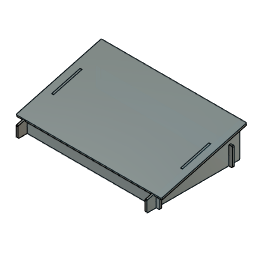
Laptop Stand (Autodesk Fusion 360 design; units mm, degrees)
Autodesk Fusion 360 part; units mm, degrees
sketch "Sketch1" plane through (0, 0, 0) normal (1, 0, 0) x (0, 1, 0) in component "Leg"
  line L0 (0, 0) -> (252.4348, 0)
  line L1 (252.4348, 0) -> (252.4348, 92.1166)
  line L2 (20.6126, 30) -> (19.3185, 34.8296)
  line L3 (19.3185, 34.8296) -> (0, 29.6532)
  line L4 (0, 29.6532) -> (0, 0)
  line L5 (97.8867, 50.7055) -> (96.5926, 55.5352)
  line L6 (96.5926, 55.5352) -> (173.8666, 76.2407)
  line L7 (173.8666, 76.2407) -> (175.1607, 71.411)
  line L8 (252.4348, 92.1166) -> (175.1607, 71.411)
  line L9 (97.8867, 50.7055) -> (20.6126, 30)
  dimension "d4" = 15
  dimension "d5" = 240
  dimension "d6" = 20
  dimension "d8" = 30
  dimension "d9" = 5
  dimension "d17" = 5
  dimension "d18" = 80
  dimension "d19" = 80
  constraint coincident L0.start L4.end
  constraint horizontal L0
  constraint perpendicular L0 L1
  constraint perpendicular L2 L8
  constraint perpendicular L0 L4
  constraint parallel L3 L8
  constraint coincident L5.start L8
  constraint perpendicular L5 L8
  constraint perpendicular L5 L6
  constraint perpendicular L7 L8
  constraint collinear L8 L9
  measures "d4" angle of L0 L8
  measures "d5" distance of L1.end L2.start
  measures "d6" distance of L2.end L3.end
  measures "d8" distance of L0 L2.start
  measures "d9" distance of L2.start L2.end
  measures "d17" distance of L5.start L5.end
  measures "d18" distance of L2 L5
  measures "d19" distance of L5.end L6.end
extrude "Extrude1" add sketch "Sketch1" along normal blind 5 makes body 1 in component "Leg"
sketch "Sketch1 (2)" plane through (0, -6.1192, 22.8372) normal (0, -0.258819, 0.965926) x (1, 0, 0) in component "Top"
  line L0 (0, 107.6748) -> (0, 27.6748)
  line L1 (0, 27.6748) -> (5, 27.6748)
  line L2 (5, 27.6748) -> (5, 107.6748)
  line L3 (5, 267.6748) -> (0, 267.6748)
  line L4 (350, 107.6748) -> (350, 27.6748)
  line L5 (350, 27.6748) -> (355, 27.6748)
  line L6 (355, 27.6748) -> (355, 107.6748)
  line L7 (355, 267.6748) -> (350, 267.6748)
  line L8 (-20, 267.6748) -> (375, 267.6748)
  line L9 (375, 267.6748) -> (375, 27.6748)
  line L10 (375, 27.6748) -> (-20, 27.6748)
  line L11 (-20, 27.6748) -> (-20, 267.6748)
  line L12 (5, 107.6748) -> (0, 107.6748)
  line L13 (0, 267.6748) -> (0, 187.6748)
  line L14 (0, 187.6748) -> (5, 187.6748)
  line L15 (5, 187.6748) -> (5, 267.6748)
  line L16 (355, 107.6748) -> (350, 107.6748)
  line L17 (350, 267.6748) -> (350, 187.6748)
  line L18 (350, 187.6748) -> (355, 187.6748)
  line L19 (355, 187.6748) -> (355, 267.6748)
  dimension "d20" = 20
  dimension "d21" = 20
  dimension "d22" = 240
  constraint horizontal L8
  constraint vertical L9
  constraint horizontal L10
  constraint vertical L11
  measures "d20" distance of L0 L11
  measures "d21" distance of L6 L9
  measures "d22" distance of L8.end L9.end
extrude "Extrude1'" add sketch "Sketch1 (2)" along normal blind 5 separate body makes body 2 in component "Top"
combine "Combine1" operation cut target body 2 tool bodies 1 1 body 1 seen with x (1, 0, 0) y (0, 1, 0) z (0, 0, 1) at (0, 0, 0) body 1 seen with x (1, 0, 0) y (0, 1, 0) z (0, 0, 1) at (350, 0, 0) keep tools in component "Top"
ref_plane "WorkPlane1" through (352.5, 25, 14.8266) normal (0, -1, 0) x (0, 0, -1) in component "support front"
sketch "Sketch1 (3)" plane through (352.5, 25, 14.8266) normal (0, -1, 0) x (1, 0, 0) in component "support front"
  line L0 (2.5, 16.349) -> (-2.5, 16.349)
  line L1 (-2.5, 16.349) -> (-2.5, -14.8266)
  line L2 (-2.5, -14.8266) -> (2.5, -14.8266)
  line L3 (2.5, -14.8266) -> (2.5, 16.349)
  line L4 (-347.5, 16.349) -> (-352.5, 16.349)
  line L5 (-352.5, 16.349) -> (-352.5, -14.8266)
  line L6 (-352.5, -14.8266) -> (-347.5, -14.8266)
  line L7 (-347.5, -14.8266) -> (-347.5, 16.349)
  line L8 (-362.5, 15.1734) -> (12.5, 15.1734)
  line L9 (12.5, 15.1734) -> (12.5, -14.8266)
  line L10 (12.5, -14.8266) -> (-362.5, -14.8266)
  line L11 (-362.5, -14.8266) -> (-362.5, 15.1734)
  line L12 (-362.5, 0.1734) -> (12.5, 0.1734)
  dimension "d26" = 10
  dimension "d27" = 10
  dimension "d29" = 30
  constraint horizontal L8
  constraint vertical L9
  constraint horizontal L10
  constraint vertical L11
  constraint collinear L6 L10
  constraint midpoint L11 L12.start
  constraint midpoint L9 L12.end
  measures "d26" distance of L5 L11
  measures "d27" distance of L3 L9
  measures "d29" distance of L8 L10
extrude "Extrude1''" add sketch "Sketch1 (3)" against normal blind 5 separate body contours L3 L8 L9 L12 | L1 L7 L8 L12 | L3 L9 L10 L12 | L1 L2 L3 L10 L12 | L1 L7 L10 L12 | L5 L6 L7 L10 L12 | L5 L8 L11 L12 | L5 L10 L11 L12 makes body 3 in component "support front"
ref_plane "WorkPlane1" through (352.5, 227.4348, 46.0583) normal (0, 1, 0) x (0, 0, 1) in component "support back"
sketch "Sketch1 (4)" plane through (352.5, 227.4348, 46.0583) normal (0, 1, 0) x (1, 0, 0) in component "support back"
  line L0 (-347.5, 46.0583) -> (-352.5, 46.0583)
  line L1 (-352.5, 46.0583) -> (-352.5, -39.3596)
  line L2 (-352.5, -39.3596) -> (-347.5, -39.3596)
  line L3 (-347.5, -39.3596) -> (-347.5, 46.0583)
  line L4 (2.5, 46.0583) -> (-2.5, 46.0583)
  line L5 (-2.5, 46.0583) -> (-2.5, -39.3596)
  line L6 (-2.5, -39.3596) -> (2.5, -39.3596)
  line L7 (2.5, -39.3596) -> (2.5, 46.0583)
  line L8 (12.5, -3.9417) -> (-362.5, -3.9417)
  line L9 (-362.5, -3.9417) -> (-362.5, 46.0583)
  line L10 (-362.5, 46.0583) -> (12.5, 46.0583)
  line L11 (12.5, 46.0583) -> (12.5, -3.9417)
  line L12 (12.5, 21.0583) -> (-362.5, 21.0583)
  dimension "d33" = 10
  dimension "d34" = 10
  dimension "d35" = 50
  constraint horizontal L8
  constraint vertical L9
  constraint horizontal L10
  constraint vertical L11
  constraint collinear L4 L10
  constraint midpoint L11 L12.start
  constraint midpoint L9 L12.end
  measures "d33" distance of L7 L11
  measures "d34" distance of L1 L9
  measures "d35" distance of L8 L10
extrude "Extrude1'''" add sketch "Sketch1 (4)" against normal blind 5 separate body contours L0 L1 L3 L10 L12 | L3 L5 L10 L12 | L1 L9 L10 L12 | L3 L5 L8 L12 | L4 L5 L7 L10 L12 | L1 L8 L9 L12 | L7 L10 L11 L12 | L7 L8 L11 L12 makes body 4 in component "support back"
combine "Combine1'" operation cut target body 1 tool bodies 3 4 body 3 seen with x (1, 0, 0) y (0, 1, 0) z (0, 0, 1) at (-350, 0, 0) body 4 seen with x (1, 0, 0) y (0, 1, 0) z (0, 0, 1) at (-350, 0, 0) keep tools in component "Leg"
fillet "Fillet1" radius 0.5 3 edges at (2.5, 96.5926, 55.5352) (2.5, 19.3185, 34.8296) (2.5, 173.8666, 76.2407) on bodies 1 in component "Leg"
fillet "Fillet1'" radius 2 4 edges at (-20, 19.9656, 32.4148) (375, 19.9656, 32.4148) (375, 251.7878, 94.5314) (-20, 251.7878, 94.5314) on bodies 2 in component "Top"
fillet "Fillet1''" radius 2 4 edges at (365, 27.5, 30) (365, 27.5, 0) (-10, 27.5, 30) (-10, 27.5, 0) on bodies 3 in component "support front"
fillet "Fillet1'''" radius 2 4 edges at (-10, 224.9348, 50) (-10, 224.9348, 0) (365, 224.9348, 50) (365, 224.9348, 0) on bodies 4 in component "support back"
fillet "Fillet2" radius 0.5 4 edges at (2.5, 25, 0) (2.5, 30, 0) (2.5, 222.4348, 0) (2.5, 227.4348, 0) on bodies 1 in component "Leg"
fillet "Fillet2'" radius 0.5 4 edges at (355, 27.5, 30) (350, 27.5, 30) (5, 27.5, 30) (0, 27.5, 30) on bodies 3 in component "support front"
fillet "Fillet2''" radius 0.5 4 edges at (355, 224.9348, 50) (350, 224.9348, 50) (5, 224.9348, 50) (0, 224.9348, 50) on bodies 4 in component "support back"
fillet "Fillet3" radius 2 4 edges at (2.5, 0, 29.6532) (2.5, 252.4348, 92.1166) (2.5, 252.4348, 0) (2.5, 0, 0) on bodies 1 in component "Leg"
sketch "top dxf" plane through (0, -7.4133, 27.6669) normal (0, -0.258819, 0.965926) x (1, 0, 0)
  arc A0 (-18, 267.6748) -> (-20, 265.6748) centre (-18, 265.6748) ccw
  line L0 (-20, 265.6748) -> (-20, 29.6748)
  arc A1 (-20, 29.6748) -> (-18, 27.6748) centre (-18, 29.6748) ccw
  line L1 (-18, 27.6748) -> (373, 27.6748)
  arc A2 (373, 27.6748) -> (375, 29.6748) centre (373, 29.6748) ccw
  line L2 (375, 29.6748) -> (375, 265.6748)
  arc A3 (375, 265.6748) -> (373, 267.6748) centre (373, 265.6748) ccw
  line L3 (373, 267.6748) -> (-18, 267.6748)
  line L4 (355, 107.6748) -> (350, 107.6748)
  line L5 (350, 107.6748) -> (350, 187.6748)
  line L6 (350, 187.6748) -> (355, 187.6748)
  line L7 (355, 187.6748) -> (355, 107.6748)
  line L8 (5, 107.6748) -> (0, 107.6748)
  line L9 (0, 107.6748) -> (0, 187.6748)
  line L10 (0, 187.6748) -> (5, 187.6748)
  line L11 (5, 187.6748) -> (5, 107.6748)
sketch "side dxf" plane through (355, 0, 0) normal (1, 0, 0) x (0, 1, 0)
  arc A0 (0, 2) -> (2, 0) centre (2, 2) ccw
  line L0 (2, 0) -> (24.5, 0)
  arc A1 (24.5, 0) -> (25, 0.5) centre (24.5, 0.5) ccw
  line L1 (25, 0.5) -> (25, 15)
  line L2 (25, 15) -> (30, 15)
  line L3 (30, 15) -> (30, 0.5)
  arc A2 (30, 0.5) -> (30.5, 0) centre (30.5, 0.5) ccw
  line L4 (30.5, 0) -> (221.9348, 0)
  arc A3 (221.9348, 0) -> (222.4348, 0.5) centre (221.9348, 0.5) ccw
  line L5 (222.4348, 0.5) -> (222.4348, 25)
  line L6 (222.4348, 25) -> (227.4348, 25)
  line L7 (227.4348, 25) -> (227.4348, 0.5)
  arc A4 (227.4348, 0.5) -> (227.9348, 0) centre (227.9348, 0.5) ccw
  line L8 (227.9348, 0) -> (250.4348, 0)
  arc A5 (250.4348, 0) -> (252.4348, 2) centre (250.4348, 2) ccw
  line L9 (252.4348, 2) -> (252.4348, 89.5101)
  arc A6 (252.4348, 89.5101) -> (249.9172, 91.442) centre (250.4348, 89.5101) ccw
  line L10 (249.9172, 91.442) -> (175.1607, 71.411)
  line L11 (175.1607, 71.411) -> (173.9961, 75.7577)
  arc A7 (173.9961, 75.7577) -> (173.3837, 76.1113) centre (173.5131, 75.6283) ccw
  line L12 (173.3837, 76.1113) -> (97.0755, 55.6646)
  arc A8 (97.0755, 55.6646) -> (96.722, 55.0522) centre (97.205, 55.1816) ccw
  line L13 (96.722, 55.0522) -> (97.8867, 50.7055)
  line L14 (97.8867, 50.7055) -> (20.6126, 30)
  line L15 (20.6126, 30) -> (19.4479, 34.3467)
  arc A9 (19.4479, 34.3467) -> (18.8356, 34.7002) centre (18.965, 34.2173) ccw
  line L16 (18.8356, 34.7002) -> (1.4824, 30.0504)
  arc A10 (1.4824, 30.0504) -> (0, 28.1186) centre (2, 28.1186) ccw
  line L17 (0, 28.1186) -> (0, 2)
sketch "front support dxf" plane through (0, 25, 0) normal (0, -1, 0) x (1, 0, 0)
  arc A0 (0, 29.5) -> (-0.5, 30) centre (-0.5, 29.5) ccw
  line L0 (-0.5, 30) -> (-8, 30)
  arc A1 (-8, 30) -> (-10, 28) centre (-8, 28) ccw
  line L1 (-10, 28) -> (-10, 2)
  arc A2 (-10, 2) -> (-8, 0) centre (-8, 2) ccw
  line L2 (-8, 0) -> (363, 0)
  arc A3 (363, 0) -> (365, 2) centre (363, 2) ccw
  line L3 (365, 2) -> (365, 28)
  arc A4 (365, 28) -> (363, 30) centre (363, 28) ccw
  line L4 (363, 30) -> (355.5, 30)
  arc A5 (355.5, 30) -> (355, 29.5) centre (355.5, 29.5) ccw
  line L5 (355, 29.5) -> (355, 15)
  line L6 (355, 15) -> (350, 15)
  line L7 (350, 15) -> (350, 29.5)
  arc A6 (350, 29.5) -> (349.5, 30) centre (349.5, 29.5) ccw
  line L8 (349.5, 30) -> (5.5, 30)
  arc A7 (5.5, 30) -> (5, 29.5) centre (5.5, 29.5) ccw
  line L9 (5, 29.5) -> (5, 15)
  line L10 (5, 15) -> (0, 15)
  line L11 (0, 15) -> (0, 29.5)
sketch "back support dxf" plane through (0, 227.4348, 0) normal (0, 1, 0) x (-1, 0, 0)
  arc A0 (0.5, 50) -> (0, 49.5) centre (0.5, 49.5) ccw
  line L0 (0, 49.5) -> (0, 25)
  line L1 (0, 25) -> (-5, 25)
  line L2 (-5, 25) -> (-5, 49.5)
  arc A1 (-5, 49.5) -> (-5.5, 50) centre (-5.5, 49.5) ccw
  line L3 (-5.5, 50) -> (-349.5, 50)
  arc A2 (-349.5, 50) -> (-350, 49.5) centre (-349.5, 49.5) ccw
  line L4 (-350, 49.5) -> (-350, 25)
  line L5 (-350, 25) -> (-355, 25)
  line L6 (-355, 25) -> (-355, 49.5)
  arc A3 (-355, 49.5) -> (-355.5, 50) centre (-355.5, 49.5) ccw
  line L7 (-355.5, 50) -> (-363, 50)
  arc A4 (-363, 50) -> (-365, 48) centre (-363, 48) ccw
  line L8 (-365, 48) -> (-365, 2)
  arc A5 (-365, 2) -> (-363, 0) centre (-363, 2) ccw
  line L9 (-363, 0) -> (8, 0)
  arc A6 (8, 0) -> (10, 2) centre (8, 2) ccw
  line L10 (10, 2) -> (10, 48)
  arc A7 (10, 48) -> (8, 50) centre (8, 48) ccw
  line L11 (8, 50) -> (0.5, 50)
sketch "Sketch1 (5)" plane through (0, -6.1192, 22.8372) normal (0, -0.258819, 0.965926) x (1, 0, 0)
  line L0 (0, 267.6748) -> (0, 27.6748)
  line L1 (0, 27.6748) -> (5, 27.6748)
  line L2 (5, 27.6748) -> (5, 267.6748)
  line L3 (5, 267.6748) -> (0, 267.6748)
  line L4 (350, 267.6748) -> (350, 27.6748)
  line L5 (350, 27.6748) -> (355, 27.6748)
  line L6 (355, 27.6748) -> (355, 267.6748)
  line L7 (355, 267.6748) -> (350, 267.6748)
  line L8 (-20, 267.6748) -> (375, 267.6748)
  line L9 (375, 267.6748) -> (375, 27.6748)
  line L10 (375, 27.6748) -> (-20, 27.6748)
  line L11 (-20, 27.6748) -> (-20, 267.6748)
  dimension "d12" = 20
  dimension "d13" = 20
  constraint horizontal L8
  constraint vertical L9
  constraint horizontal L10
  constraint vertical L11
  constraint collinear L7 L8
  constraint collinear L5 L10
  measures "d12" distance of L0 L11
  measures "d13" distance of L6 L9
sketch "Sketch2" plane through (0, -6.1192, 22.8372) normal (0, -0.258819, 0.965926) x (1, 0, 0)
  line L0 (0, 267.6748) -> (0, 27.6748)
  line L1 (0, 27.6748) -> (5, 27.6748)
  line L2 (5, 27.6748) -> (5, 267.6748)
  line L3 (5, 267.6748) -> (0, 267.6748)
component "Leg" placed x (1, 0, 0) y (0, 1, 0) z (0, 0, 1) at (0, 0, 0)
component "Leg" placed x (1, 0, 0) y (0, 1, 0) z (0, 0, 1) at (350, 0, 0)
component "Top" placed x (1, 0, 0) y (0, 1, 0) z (0, 0, 1) at (0, 0, 0)
component "support front" placed x (1, 0, 0) y (0, 1, 0) z (0, 0, 1) at (0, 0, 0)
component "support back" placed x (1, 0, 0) y (0, 1, 0) z (0, 0, 1) at (0, 0, 0)
equation "width = 240 mm"
equation "thickness = 5 mm"
equation "length = 350 mm"
equation "d5 = width"
equation "d9 = thickness"
equation "d10 = thickness"
equation "flange = 80 mm"
equation "d17 = thickness"
equation "d18 = flange"
equation "d19 = flange"
equation "d22 = width"
equation "d23 = thickness"
equation "d30 = -thickness"
equation "d36 = -thickness"
